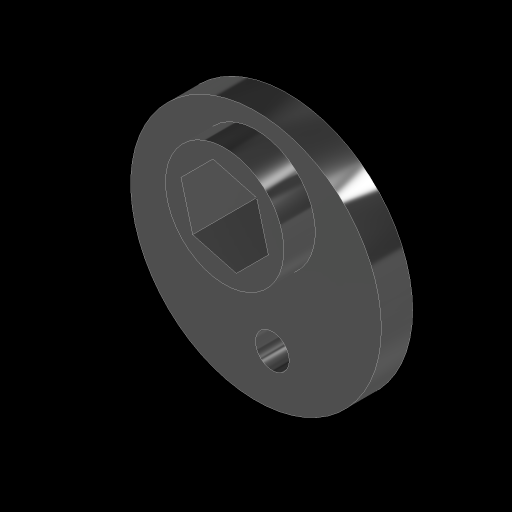
# Autodesk Inventor part: ShufflerMidCam
Saved by Autodesk Inventor 2023 (Build 270158000, 158)
## iProperties
Created: 2022-03-06
Part Number: ShufflerMidCam
Material: Custom TPU
Document SubType Name: Modeling
Designer: tandu
Density: 1.21 g/cm^3
Appearance: Smoked - Light
Mass: 1.22563 g
Surface Area: 10.5217 cm^2
Volume: 1.01292 cm^3
Author: tandu
Autodesk Inventor part; units mm, degrees
ref_plane "YZ Plane" through (0, 0, 0) normal (1, 0, 0) x (0, 1, 0)
ref_plane "XZ Plane" through (0, 0, 0) normal (0, 1, 0) x (-1, 0, 0)
ref_plane "XY Plane" through (0, 0, 0) normal (0, 0, 1) x (1, 0, 0)
sketch "Sketch1" plane through (0, 0, 0) normal (0, 0, 1) x (1, 0, 0)
  line L0 (27.0399, -21.1099) -> (29.2899, -19.8109)
  line L1 (27.0399, -23.708) -> (27.0399, -21.1099)
  line L2 (29.2899, -19.8109) -> (31.5399, -21.1099)
  line L3 (31.5399, -21.1099) -> (31.5399, -23.708)
  line L4 (29.2899, -25.007) -> (27.0399, -23.708)
  line L5 (31.5399, -23.708) -> (29.2899, -25.007)
  line L6 (31.5399, -23.708) -> (27.0399, -21.1099) construction
  line L7 (31.5399, -21.1099) -> (27.0399, -23.708) construction
  line L8 (29.2899, -25.007) -> (29.2899, -19.8109) construction
  line L9 (-3.9688, 2.2914) -> (0, 4.5827) construction
  line L10 (-3.9688, -2.2914) -> (-3.9688, 2.2914) construction
  line L11 (0, 4.5827) -> (3.9688, 2.2914) construction
  line L12 (3.9688, 2.2914) -> (3.9688, -2.2914) construction
  line L13 (0, -4.5827) -> (-3.9688, -2.2914) construction
  line L14 (3.9688, -2.2914) -> (0, -4.5827) construction
  line L15 (3.9688, -2.2914) -> (-3.9688, 2.2914) construction
  line L16 (3.9688, 2.2914) -> (-3.9688, -2.2914) construction
  line L17 (0, -4.5827) -> (0, 4.5827) construction
  line L18 (0, 0) -> (7.8286, 0) construction
  line L19 (0, 0) -> (1.6577, -12.5913) construction
  circle A0 centre (1.6577, -12.5913) radius 1.7145
  circle A1 centre (0, -5.08) radius 12.7
  line L20 (0, -5.08) -> (0, 0) construction
  line L21 (0, 0) -> (-1.6577, -12.5913) construction
  circle A2 centre (-1.6577, -12.5913) radius 1.7145
  circle A3 centre (0, 0) radius 6
  line L22 (4.4266, -1.1861) -> (1.1861, -4.4266)
  line L23 (-1.1861, 4.4266) -> (3.2405, 3.2405)
  line L24 (-4.4266, 1.1861) -> (-1.1861, 4.4266)
  line L25 (-3.2405, -3.2405) -> (-4.4266, 1.1861)
  line L26 (1.1861, -4.4266) -> (-3.2405, -3.2405)
  line L27 (3.2405, 3.2405) -> (4.4266, -1.1861)
  point P0 (29.2899, -22.4089)
  dimension "d2" = 60
  dimension "d3" = 4.5
  dimension "d4" = 60
  dimension "d5" = 7.9375
  dimension "d8" = 12.7
  dimension "d9" = 3.429
  dimension "d10" = 25.4
  dimension "d11" = 5.08
  dimension "d12" = 7.5
  dimension "d18" = 12
  dimension "d21" = 7.5
  dimension "d24" = 15
  constraints: 56 end point, 11 equal length, 4 centre point, 4 coincident, 4 parallel, 4 vertical, 3 horizontal alignment, 2 midpoint, 1 equal radius, 1 horizontal, 1 vertical alignment, 13 other
  measures "d2" angle of L3 L2
  measures "d3" distance between parallel lines of L1 L3
  measures "d4" angle of L12 L11
  measures "d5" distance between parallel lines of L10 L12
  measures "d8" distance of L18.start L19.end
  measures "d9" diameter of A0
  measures "d10" diameter of A1
  measures "d11" distance of L20.start L18.start
  measures "d12" angle of L17 L21
  measures "d18" diameter of A3
  measures "d21" angle of L19 L20
extrude "Base" add sketch "Sketch1" along normal blind 3.175 contours A0 A2 | A1 | A3 picked at (-2.2485, -12.7764)
extrude "Extrusion3" add sketch "Sketch1" along normal blind 3.175 from surface at 3.175 contours A3
equation "\"d5\" = HexSize"
equation "\"d8\" = NubOffset"
equation "\"d10\" = CamSize1"
equation "\"d11\" = Offset1"
equation "\"d12\" = NubAngle1"
equation "\"d18\" = EndCamBearingID"
equation "\"d21\" = NubAngle1"
equation "\"d24\" = 2 * NubAngle1"
equation "\"HexSize\" = 7.9375"
equation "\"NubOffset\" = 12.7"
equation "\"CamSize1\" = 25.4"
equation "\"Offset1\" = 5.08"
equation "\"NubAngle1\" = 7.5deg"
equation "\"EndCamBearingID\" = 12"
body "Solid1"
